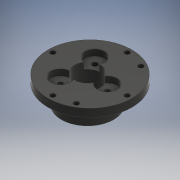
# Autodesk Inventor part: AC10
Saved by Autodesk Inventor 2017 (Build 210142000, 142)
## iProperties
Created: 2019-11-04
Part Number: AC10
Material: ABS Plastic
Document SubType Name: Modeling
Designer: Dell
Density: 1.06 g/cm^3
Appearance: Smooth - Black
Author: Dell
Autodesk Inventor part; units mm, degrees
ref_plane "YZ Plane" through (0, 0, 0) normal (1, 0, 0) x (0, 1, 0)
ref_plane "XZ Plane" through (0, 0, 0) normal (0, 1, 0) x (-1, 0, 0)
ref_plane "XY Plane" through (0, 0, 0) normal (0, 0, 1) x (1, 0, 0)
sketch "Sketch1" plane through (0, 0, 0) normal (0, 0, 1) x (1, 0, 0)
  circle A0 centre (0, 0) radius 33
  circle A1 centre (0, 0) radius 16.5
  circle A2 centre (25, 0) radius 3.5
  circle A3 centre (-12.5, 21.6506) radius 3.5
  circle A4 centre (-12.5, -21.6506) radius 3.5
  dimension "d0" = 66
  dimension "d1" = 33
  dimension "d2" = 7
  dimension "d3" = 25
  dimension "d6" = 360
  constraints: 5 centre point, 2 coincident, 1 horizontal alignment, 7 other
  measures "d0" diameter of A0
  measures "d1" diameter of A1
  measures "d2" diameter of A2
  measures "d3" distance of point (0, 0) A2.centre
extrude "Extrusion1" add sketch "Sketch1" along normal blind 35
sketch "Sketch3" plane through (0, 0, 35) normal (0, 0, 1) x (1, 0, 0)
  circle A0 centre (3.125, 0) radius 53
  circle A1 centre (0, 0) radius 10
  circle A2 centre (26.625, -40.7032) radius 3.15
  circle A3 centre (18.75, 0) radius 5.5
  circle A4 centre (50.125, 0) radius 3.15
  circle A5 centre (26.625, 40.7032) radius 3.15
  circle A6 centre (3.125, -47) radius 3.15
  circle A7 centre (3.125, 47) radius 3.15
  circle A8 centre (-43.875, 0) radius 3.15
  line L0 (3.125, 0) -> (3.125, 47)
  line L1 (3.125, 0) -> (26.625, 40.7032)
  line L2 (3.125, 0) -> (50.125, 0)
  line L3 (26.625, -40.7032) -> (3.125, 0)
  line L4 (3.125, 0) -> (3.125, -47)
  line L5 (3.125, 0) -> (-43.875, 0)
  circle A9 centre (0, 0) radius 33 projected
  point P0 (0, 0)
  dimension "d19" = 106
  dimension "d20" = 6.3
  dimension "d21" = 6.3
  dimension "d22" = 6.3
  dimension "d23" = 6.3
  dimension "d24" = 6.3
  dimension "d25" = 6.3
  dimension "d27" = 20
  dimension "d28" = 18.75
  dimension "d35" = 30
  dimension "d36" = 30
  dimension "d37" = 3.125
  dimension "d38" = 11
  dimension "d41" = 47
  dimension "d44" = 47
  dimension "d45" = 47
  dimension "d46" = 47
  dimension "d47" = 47
  dimension "d48" = 47
  constraints: 12 end point, 9 centre point, 2 coincident, 2 perpendicular, 2 point on line, 1 collinear, 1 horizontal
  measures "d19" diameter of A0
  measures "d20" diameter of A8
  measures "d21" diameter of A7
  measures "d22" diameter of A5
  measures "d23" diameter of A4
  measures "d24" diameter of A2
  measures "d25" diameter of A6
  measures "d27" diameter of A1
  measures "d28" distance of point (0, 0) A3.centre
  measures "d35" angle of L0 L1
  measures "d36" angle of L4 L3
  measures "d37" distance of A1.centre L0.start
  measures "d38" diameter of A3
  measures "d41" distance of L5.end L0.start
  measures "d44" distance of L2.end L0.start
  measures "d45" distance of L0.start L0.end
  measures "d46" distance of L0.start L4.end
  measures "d47" distance of L3.start L0.start
  measures "d48" distance of L0.start L1.end
extrude "Extrusion4" add sketch "Sketch3" against normal blind 10
sketch "Sketch4" plane through (3.125, 0, 35) normal (0, 0, 1) x (1, 0, 0)
  circle A0 centre (18.75, 0) radius 7.5
  point P0 (-3.125, 0)
  dimension "d49" = 15
  dimension "d50" = 21.875
  constraints: 1 centre point, 1 horizontal alignment
  measures "d49" diameter of A0
  measures "d50" distance of A0.centre point (-3.125, 0)
extrude "Extrusion5" cut sketch "Sketch4" against normal blind 5
sketch "Sketch5" plane through (3.125, 0, 35) normal (0, 0, 1) x (1, 0, 0)
  circle A0 centre (21.875, 0) radius 3.5 projected
  circle A1 centre (21.875, 0) radius 3.5 projected
  circle A2 centre (21.875, 0) radius 12.5
  circle A3 centre (-15.625, 21.6506) radius 12.5
  circle A4 centre (-15.625, -21.6506) radius 12.5
  point P0 (-3.125, 0)
  dimension "d53" = 25
  dimension "d56" = 360
  constraints: 3 centre point, 1 coincident, 7 other
  measures "d53" diameter of A2
extrude "Extrusion6" cut sketch "Sketch5" against normal blind 8 contours A0 | A2 | A3 | A4
body "Solid1"
